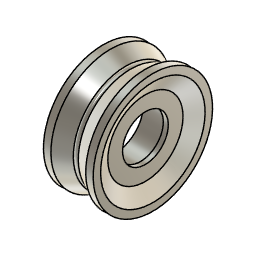
side_pulley v5 (Autodesk Fusion 360 design; units mm, degrees)
Autodesk Fusion 360 part; units mm, degrees
sketch "Sketch1" plane through (0, 0, 0) normal (0, 1, 0) x (1, 0, 0)
  line L0 (0, 0) -> (5, 0)
  line L1 (5, 0) -> (5, -10.5)
  line L2 (5, -10.5) -> (0, -10.5)
  line L3 (0, -10.5) -> (0, 0)
  line L4 (5, -10.5) -> (5, -12)
  line L5 (5, -12) -> (3.5, -12)
  circle A0 centre (0, -10.5) radius 0.5
  line L6 (3.5, -12) -> (0.5, -10.5)
  line L7 (0, 0) -> (0, -5.6)
  line L8 (0, -5.6) -> (2.5, -5.6)
  line L9 (2.5, -5.6) -> (5, -10.5)
  point P0 (0, -10)
  dimension "d1" = 5
  dimension "d2" = 10.5
  dimension "d3" = 1
  dimension "d7" = 1.5
  dimension "d8" = 1.5
  dimension "d9" = 5.6
  dimension "d10" = 2.5
  constraint horizontal L0
  constraint vertical L1
  constraint horizontal L2
  constraint vertical L3
  constraint coincident L0.start L3.end
  constraint perpendicular L2 L4
  constraint perpendicular L4 L5
  constraint coincident L2.end L3.start
  constraint coincident A0 L6.end
  constraint coincident L2 L6.end
  constraint perpendicular L0 L7
  constraint perpendicular L3 L8
  constraint coincident A0 P0
  constraint coincident L3 P0
  measures "d1" distance of L0.start L0.end
  measures "d2" distance of L0.start L2.end
  measures "d3" diameter of A0
  measures "d7" distance of L1.end L4.end
  measures "d8" distance of L4.end L5.end
  measures "d9" distance of L0.start L7.end
  measures "d10" distance of L7.end L8.end
revolve "Revolve1" add sketch "Sketch1" angle 360 about axis through (1.75, 0, 0) along (1, 0, 0) contours L2 L3 A0 L8 L9 | L2 L4 L5 L6
mirror "Mirror1" about plane through (0, 0, 0) normal (1, 0, 0) of bodies 1 merged
sketch "Sketch2" plane through (0, 0, 0) normal (0, 1, 0) x (1, 0, 0)
  line L0 (0, 0) -> (5, 0)
  line L1 (5, 0) -> (5, -10.5)
  line L2 (2.5, 0) -> (2.5, -5.6)
  line L3 (5, -10.5) -> (2.5, -5.6)
  line L4 (3.5, 0) -> (3.5, -7.56)
  line L5 (2.5, -4.6) -> (3.5, -4.6)
  dimension "d11" = 10.5
  dimension "d12" = 5.6
  dimension "d13" = 1
  dimension "d14" = 1
  constraint coincident L0.start origin
  constraint horizontal L0
  constraint perpendicular L0 L1
  constraint midpoint L0 L2.start
  constraint perpendicular L0 L2
  constraint coincident L0 L4.start
  constraint coincident L3 L4.end
  constraint perpendicular L0 L4
  constraint coincident L2 L5.start
  constraint coincident L4 L5.end
  constraint perpendicular L4 L5
  measures "d11" distance of L0.end L1.end
  measures "d12" distance of L2.start L2.end
  measures "d13" distance of L2 L4
  measures "d14" distance of L2.end L5
revolve "Revolve2" add sketch "Sketch2" angle 360 about axis through (0, 0, 0) along (1, 0, 0) contours L2 L3 L4 L5
